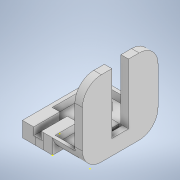
# Autodesk Inventor part: InstaMeter
Saved by Autodesk Inventor 2020 (Build 240168000, 168)
## iProperties
Created: 2020-01-07
Part Number: InstaMeter
Material: Générique
Document SubType Name: Modeling
Designer: laura
Density: 1 g/cm^3
Appearance: Par défaut
Author: laura
## iProperties of the stored document _Impression 3D.ipt
Created: 2020-01-09
Part Number: _Impression 3D
Material: Générique
Document SubType Name: Modeling
Designer: laura
Density: 1 g/cm^3
Appearance: Par défaut
Author: laura
Autodesk Inventor part; units mm, degrees
ref_plane "YZ Plane" through (0, 0, 0) normal (1, 0, 0) x (0, 1, 0)
sketch "Esquisse1" plane through (0, 0, 0) normal (0, 1, 0) x (-1, 0, 0)
  line L0 (0, 0) -> (-40, 0)
  line L1 (-40, 0) -> (-40, -80)
  line L2 (-40, -80) -> (0, -80)
  line L3 (0, -80) -> (0, 0)
  dimension "d0" = 80
  dimension "d4" = 40
  constraints: 8 end point, 2 parallel, 1 horizontal, 1 perpendicular
  measures "d0" distance between parallel lines of L2 L0
  measures "d4" distance between parallel lines of L1 L3
extrude "Extrusion1" add sketch "Esquisse1" along normal blind 80
sketch "Esquisse2" plane through (40, 0, 0) normal (1, 0, 0) x (0, 0, -1)
  point P0 (0, 0)
sketch "Esquisse3" plane through (40, 0, 0) normal (1, 0, 0) x (0, 0, -1)
  line L0 (0, 80) -> (80, 80) projected
  line L1 (20, 20) -> (60, 20)
  line L2 (60, 20) -> (60, 80)
  line L3 (60, 80) -> (20, 80)
  line L4 (20, 80) -> (20, 20)
  line L5 (0, 0) -> (80, 0) projected
  line L6 (80, 0) -> (80, 80) projected
  line L7 (0, 0) -> (0, 80) projected
  point P0 (20, 80)
  dimension "d9" = 20
  dimension "d10" = 20
  dimension "d11" = 20
  constraints: 8 end point, 2 parallel, 1 horizontal, 1 perpendicular, 1 point on line
  measures "d9" distance between parallel lines of L5 L1
  measures "d10" distance between parallel lines of L6 L2
  measures "d11" distance between parallel lines of L7 L4
extrude "Extrusion2" cut sketch "Esquisse3" against normal blind 80 contours L0 L2 L1 L4
sketch "Esquisse4" plane through (40, 20, -20) normal (0, 1, 0) x (1, 0, 0)
  line L0 (0, 40) -> (-40, 40) projected
  line L1 (0, 0) -> (-5, 0)
  line L2 (-5, 40) -> (0, 40)
  line L3 (0, 40) -> (0, 0)
  line L4 (-5, 40) -> (-10, 40)
  line L5 (-9, 10) -> (-12, 10)
  line L6 (-12, 10) -> (-12, 30)
  line L7 (-12, 30) -> (-9, 30)
  line L8 (-9, 10) -> (-9, 30)
  point P0 (-40, -20)
  dimension "d19" = 20
  dimension "d21" = 9
  dimension "d22" = 3
  constraints: 16 end point, 2 horizontal, 2 vertical, 1 parallel, 1 point on line
  measures "d19" distance of L5.end L6.end
  measures "d21" distance between parallel lines of L8 L3
  measures "d22" distance of L5.start L5.end
extrude "Extrusion3" cut sketch "Esquisse4" against normal blind 10
sketch "Esquisse6" plane through (40, 20, -20) normal (0, 0, -1) x (-1, 0, 0)
  line L0 (40, 60) -> (40, 0) projected
  line L1 (0, 60) -> (40, 60) projected
  line L2 (0, 0) -> (0, 60) projected
  line L3 (0, 0) -> (40, 0) projected
  point P0 (40, -20)
extrude "Extrusion4" add sketch "Esquisse6" along normal blind 9
sketch "Esquisse7" plane through (40, 20, -60) normal (0, 0, 1) x (1, 0, 0)
  line L0 (-40, 0) -> (-40, 60) projected
  line L1 (0, 0) -> (-40, 0) projected
  line L2 (0, 60) -> (0, 0) projected
  line L3 (-40, 60) -> (0, 60) projected
  point P0 (-40, -20)
extrude "Extrusion5" add sketch "Esquisse7" along normal blind 9
sketch "Esquisse8" plane through (0, 80, 0) normal (0, 1, 0) x (1, 0, 0)
  line L0 (40, 51) -> (40, 80) projected
  line L1 (40, 80) -> (0, 80) projected
  line L2 (0, 80) -> (0, 51) projected
  line L3 (40, 51) -> (0, 51) projected
  point P0 (0, 0)
extrude "Extrusion6" add sketch "Esquisse8" along normal blind 20
sketch "Esquisse9" plane through (0, 80, 0) normal (0, 1, 0) x (1, 0, 0)
  line L0 (0, 29) -> (0, 0) projected
  line L1 (0, 0) -> (40, 0) projected
  line L2 (40, 0) -> (40, 29) projected
  line L3 (0, 29) -> (40, 29) projected
extrude "Extrusion7" add sketch "Esquisse9" along normal blind 20
sketch "Esquisse10" plane through (0, 0, 0) normal (0, 0, 1) x (1, 0, 0)
  line L0 (0, 0) -> (40, 0) projected
  line L1 (40, 0) -> (40, 100) projected
  line L2 (0, 100) -> (40, 100) projected
  line L3 (0, 0) -> (0, 100) projected
extrude "Extrusion8" add sketch "Esquisse10" along normal blind 10
sketch "Esquisse11" plane through (40, 0, -80) normal (0, 0, -1) x (-1, 0, 0)
  line L0 (0, 0) -> (40, 0) projected
  line L1 (40, 0) -> (40, 100) projected
  line L2 (0, 100) -> (40, 100) projected
  line L3 (0, 0) -> (0, 100) projected
extrude "Extrusion9" add sketch "Esquisse11" along normal blind 10
sketch "Esquisse12" plane through (0, 20, -51) normal (-1, 0, 0) x (0, 0, 1)
  line L0 (22, 80) -> (61, 80) projected
  line L1 (61, 80) -> (36, 80)
  line L2 (61, 80) -> (61, 55)
  line L3 (61, 80) -> (61, -20) projected
  arc A0 (61, 55) -> (36, 80) centre (36, 55) ccw
  point P0 (51, -20)
  dimension "d35" = 25
  dimension "d36" = 25
  constraints: 4 end point, 2 point on circle, 2 point on line, 1 centre point, 1 tangent
  measures "d35" distance of L0.end L1.end
  measures "d36" distance of L0.end L2.end
ref_plane "Plan de construction1" through (40, 0, -40) normal (0, 0, -1) x (-1, 0, 0)
extrude "Extrusion10" cut sketch "Esquisse12" against normal up to surface (40 mm away)
mirror "Symétrie1" about plane through (40, 0, -40) normal (0, 0, -1) of "Extrusion10"
ref_plane "Plan de construction2" through (0, 50, 0) normal (0, 1, 0) x (1, 0, 0)
mirror "Symétrie2" about plane through (0, 50, 0) normal (0, 1, 0) of "Extrusion10", "Symétrie1"
sketch "Esquisse13" plane through (0, 20, -51) normal (-1, 0, 0) x (0, 0, 1)
  line L0 (11, -10) -> (-14, -10)
  line L1 (11, -10) -> (36, -10)
  line L2 (-14, -10) -> (-14, 0)
  line L3 (-14, 0) -> (-38.4949, 0)
  line L4 (36, -10) -> (36, 0)
  line L5 (36, 0) -> (60.4949, 0)
  arc A0 (-38.4949, 0) -> (-14, -20) centre (-14, 5) ccw
  arc A1 (36, -20) -> (60.4949, 0) centre (36, 5) ccw
  line L6 (36, -20) -> (-14, -20)
  point P0 (51, -20)
  dimension "d40" = 25
  dimension "d41" = 25
  dimension "d42" = 10
  constraints: 14 end point, 4 point on circle, 2 centre point, 2 point on line
  measures "d40" distance of L0.start L0.end
  measures "d41" distance of L0.start L1.end
  measures "d42" distance of L0.end L2.end
extrude "Extrusion11" add sketch "Esquisse13" along normal blind 40
sketch "Esquisse14" plane through (0, 10, -15) normal (0, 1, 0) x (1, 0, 0)
  line L0 (-40, 0) -> (-40, 50) projected
  line L1 (-40, 0) -> (40, 0) projected
  line L2 (-40, 50) -> (-35, 50)
  line L3 (-35, 50) -> (-35, 0)
  line L4 (-35, 0) -> (-40, 0)
  line L5 (-40, 0) -> (-40, 50)
  point P0 (0, -15)
  dimension "d45" = 5
  constraints: 8 end point, 2 parallel, 1 horizontal, 1 perpendicular, 1 point on line
  measures "d45" distance of L3.end L4.end
extrude "Extrusion12" add sketch "Esquisse14" along normal up to surface (10 mm away)
sketch "Esquisse15" plane through (0, 20, 9.4949) normal (0, 1, 0) x (1, 0, 0)
  line L0 (-17.5, 24.4949) -> (-12.5, 24.4949)
  line L1 (-12.5, 24.4949) -> (-22.5, 24.4949)
  line L2 (-22.5, 24.4949) -> (-22.5, 0)
  line L3 (-12.5, 24.4949) -> (-12.5, 0)
  line L4 (-22.5, 0) -> (-12.5, 0)
  dimension "d48" = 5
  dimension "d49" = 10
  constraints: 10 end point, 2 perpendicular, 1 parallel
  measures "d48" distance of L0.start L0.end
  measures "d49" distance of L0.end L1.end
extrude "Extrusion13" cut sketch "Esquisse15" against normal up to surface (10 mm away)
sketch "Esquisse16" plane through (40, 20, -51) normal (0, 0, 1) x (1, 0, 0)
  point P0 (-40, -20)
sketch "Esquisse17" plane through (31, 20, -50) normal (-1, 0, 0) x (0, 0, 1)
  line L0 (0, 0) -> (20, 0) projected
  line L1 (0, 0) -> (0, -10) projected
  line L2 (0, -10) -> (20, -10) projected
  line L3 (20, 0) -> (20, -10) projected
  point P0 (50, -20)
extrude "Extrusion14" cut sketch "Esquisse17" against normal blind 1
sketch "Esquisse18" plane through (0, 20, -51) normal (-1, 0, 0) x (0, 0, 1)
  line L0 (22, 0) -> (22, 80)
  line L1 (22, 80) -> (36, 80)
  arc A0 (61, 55) -> (36, 80) centre (36, 55) ccw
  line L2 (-38.4949, 0) -> (-14, 0)
  line L3 (36, 0) -> (60.4949, 0)
  arc A1 (60.4949, 0) -> (61, 5) centre (36, 5) ccw
  line L4 (61, 55) -> (61, 5)
  arc A2 (61, 55) -> (36, 80) centre (36, 55) ccw
  line L5 (22, 80) -> (36, 80)
  line L6 (22, 0) -> (22, 80)
  line L7 (22, 0) -> (0, 0)
  line L8 (0, 0) -> (0, 80)
  line L9 (0, 80) -> (-14, 80)
  arc A3 (-14, 80) -> (-39, 55) centre (-14, 55) ccw
  line L10 (-39, 5) -> (-39, 55)
  arc A4 (-39, 5) -> (-38.4949, 0) centre (-14, 5) ccw
  arc A5 (-39, 5) -> (-38.4949, 0) centre (-14, 5) ccw
  line L11 (-38.4949, 0) -> (60.4949, 0)
  point P0 (51, -20)
  point P1 (61, 55)
  point P2 (22, 0)
  point P3 (36, 0)
  constraints: 24 end point, 12 point on circle, 10 centre point
extrude "Extrusion15" cut sketch "Esquisse18" against normal blind 30
sketch "Esquisse19" plane through (0, 10, -65) normal (0, 0, 1) x (1, 0, 0)
  line L0 (-35, 10) -> (-35, 0) projected
  line L1 (0, 0) -> (-35, 0) projected
  line L2 (0, 10) -> (0, 0) projected
  line L3 (0, 10) -> (-35, 10) projected
  point P0 (0, -10)
extrude "Extrusion16" cut sketch "Esquisse19" against normal blind 20
sketch "Esquisse20" plane through (0, 10, -15) normal (-1, 0, 0) x (0, 0, 1)
  arc A0 (0, -10) -> (25, 15) centre (0, 15) ccw projected
  line L0 (25, 15) -> (25, -10)
  line L1 (25, -10) -> (0, -10)
  line L2 (24.498, 10.0154) -> (25, 10.0154)
  point P0 (15, -10)
  constraints: 6 end point, 2 perpendicular, 2 tangent, 1 point on circle, 1 point on line, 1 vertical
extrude "Extrusion17" add sketch "Esquisse20" along normal up to surface (40 mm away) contours A0 L2 L0 L1
mirror "Symétrie3" about plane through (40, 0, -40) normal (0, 0, -1) of "Extrusion17"
sketch "Esquisse21" plane through (0, 0, 10) normal (0, 0, 1) x (1, 0, 0)
  line L0 (-22.5, 20) -> (-22.5, 10) projected
  line L1 (-12.5, 10) -> (-12.5, 20) projected
  line L2 (-22.5, 10) -> (-35, 10) projected
  line L3 (-12.5, 10) -> (-22.5, 10) projected
  line L4 (0, 10) -> (-12.5, 10) projected
  line L5 (-35, 10) -> (0, 10) projected
  line L6 (0, 20) -> (-12.5, 20) projected
  line L7 (-22.5, 20) -> (-22.5, 21.5856)
  line L8 (-12.5, 20) -> (-12.5, 21.5856)
  line L9 (-12.5, 21.5856) -> (-22.5, 21.5856)
  point P0 (0, 0)
  point P1 (-22.5, 10)
  point P2 (-12.5, 10)
  constraints: 6 end point, 2 vertical, 1 perpendicular
extrude "Extrusion18" cut sketch "Esquisse21" against normal blind 20
sketch "Esquisse23" plane through (40, 20, -29) normal (0, 1, 0) x (1, 0, 0)
  line L0 (-40, -14) -> (-40, 56)
  line L1 (-10, 0) -> (0, 0)
  line L2 (-8, 22) -> (-10, 22)
  line L3 (-10, 22) -> (-10, 56)
  line L4 (-8, 1) -> (-12, 1)
  line L5 (-12, 21) -> (-8, 21)
  line L6 (-8, 21) -> (-8, 1)
  line L7 (-10, 22) -> (-10, 56)
  line L8 (-10, 22) -> (-40, 22)
  line L9 (-40, -14) -> (-40, 56)
  line L10 (-10, 22) -> (-10, 56)
  line L11 (-40, 56) -> (-10, 56)
  point P0 (-10, -38.4949)
  point P1 (-40, 22)
  constraints: 24 end point, 2 point on line
extrude "Extrusion20" cut sketch "Esquisse23" against normal blind 10
mirror "Symétrie4" about plane through (40, 0, -40) normal (0, 0, -1) of "Extrusion20"
sketch "Esquisse24" plane through (0, 20, 9.4949) normal (0, 1, 0) x (1, 0, 0)
  point P0 (0, 9.4949)
sketch "Esquisse25" plane through (0, 20, 9.4949) normal (0, 1, 0) x (1, 0, 0)
  point P0 (0, 9.4949)
sketch "Esquisse26" plane through (0, 0, 10) normal (0, 0, 1) x (1, 0, 0)
  point P0 (0, 0)
sketch "Esquisse27" plane through (-40, 20.0154, 9.498) normal (0, 1, 0) x (1, 0, 0)
  line L0 (27.5, -0.502) -> (27.5, 24.498) projected
  line L1 (40, 24.498) -> (40, -0.502) projected
  line L2 (27.5, 0.0017) -> (40, 0.0017)
  line L3 (40, 0.0017) -> (40, -0.502)
  line L4 (40, -0.502) -> (27.5, -0.502)
  line L5 (27.5, -0.502) -> (27.5, 0.0017)
  point P0 (40, 9.498)
  constraints: 8 end point, 2 parallel, 1 horizontal, 1 perpendicular, 1 point on line
extrude "Extrusion21" cut sketch "Esquisse27" against normal blind 25
sketch "Esquisse28" plane through (-40, 20.0154, 9.498) normal (0, 1, 0) x (1, 0, 0)
  point P0 (40, 9.498)
sketch "Esquisse29" plane through (-40, 20.0154, 9.498) normal (0, 1, 0) x (1, 0, 0)
  line L0 (17.5, -0.502) -> (17.5, 0) projected
  line L1 (17.5, 0) -> (0, 0) projected
  line L2 (0, 0) -> (0, -0.502) projected
  line L3 (17.5, -0.502) -> (0, -0.502) projected
  point P0 (40, 9.498)
extrude "Extrusion22" cut sketch "Esquisse29" against normal up to surface (20.0154 mm away)
sketch "Esquisse30" plane through (-35, 10, -15) normal (0, 1, 0) x (1, 0, 0)
  line L0 (22.5, -25) -> (12.5, -25) projected
  line L1 (12.5, -25) -> (12.5, -24.4949)
  line L2 (22.5, -24.4963) -> (22.5, 0) projected
  line L3 (12.5, -24.4949) -> (22.5, -24.4963)
  line L4 (22.5, -25) -> (22.5, -24.4963) projected
  line L5 (22.5, -24.4963) -> (22.5, -25)
  point P0 (35, -15)
  constraints: 6 end point, 1 vertical
extrude "Extrusion23" cut sketch "Esquisse30" against normal up to surface (10 mm away)
sketch "Esquisse31" plane through (-40, 20.0154, -89.498) normal (0, 1, 0) x (1, 0, 0)
  line L0 (0, 0) -> (0, 0.502) projected
  line L1 (40, 0) -> (0, 0) projected
  line L2 (40, 0.502) -> (40, 0) projected
  line L3 (40, 0.502) -> (0, 0.502) projected
  point P0 (40, -89.498)
extrude "Extrusion24" cut sketch "Esquisse31" against normal up to surface (20.0154 mm away)
sketch "Esquisse32" plane through (0, 10, -51) normal (-1, 0, 0) x (0, 0, 1)
  line L0 (0, 0) -> (0, 10)
  line L1 (0, 10) -> (22, 10)
  line L2 (22, 10) -> (22, 0)
  line L3 (22, 0) -> (0, 0)
  point P0 (51, -10)
  constraints: 8 end point, 2 parallel, 1 perpendicular, 1 vertical
extrude "Extrusion25" add sketch "Esquisse32" along normal blind 5
sketch "Esquisse37" plane through (-35, 20, -15) normal (0, 1, 0) x (1, 0, 0)
  line L0 (12.5, 0) -> (0, 0) projected
  line L1 (12.5, 0) -> (10, 0)
  line L2 (10, 0) -> (10, -25.2265)
  line L3 (10, -25.2265) -> (12.5, -25.2265)
  line L4 (12.5, -25.2265) -> (12.5, 0)
  point P0 (35, -15)
  dimension "d78" = 2.5
  constraints: 8 end point, 2 parallel, 1 horizontal, 1 perpendicular
  measures "d78" distance of L3.end L2.end
extrude "Extrusion27" cut sketch "Esquisse37" against normal blind 10
sketch "Esquisse39" plane through (0, 20, 9.4949) normal (0, 1, 0) x (1, 0, 0)
  line L0 (-12.5, 24.4949) -> (-12.5, 0) projected
  line L1 (-12.5, 24.4949) -> (-12.5, 0)
  line L2 (-12.5, 0) -> (-15, 0)
  line L3 (-15, 0) -> (-15, 24.4949)
  line L4 (-15, 24.4949) -> (-12.5, 24.4949)
  point P0 (0, 9.4949)
  dimension "d81" = 2.5
  constraints: 8 end point, 2 parallel, 1 perpendicular, 1 vertical
  measures "d81" distance of L0.end L2.end
extrude "Extrusion28" add sketch "Esquisse39" against normal blind 10
sketch "Esquisse40" plane through (-35, 10, -15) normal (0, 1, 0) x (1, 0, 0)
  line L0 (30, 14) -> (30, 36) projected
  line L1 (30, 14) -> (30, 0)
  line L2 (35, 0) -> (20, 0) projected
  line L3 (35, -20) -> (35, 0) projected
  line L4 (35, -20) -> (35, 0)
  line L5 (35, 0) -> (30, 0)
  line L6 (30, 0) -> (30, -20)
  line L7 (30, -20) -> (35, -20)
  point P0 (35, -15)
  point P1 (30, 0)
  constraints: 10 end point, 3 equal length, 1 perpendicular, 1 point on line, 1 vertical
extrude "Extrusion29" cut sketch "Esquisse40" along normal blind 10
sketch "Esquisse41" plane through (-15, 10, -15) normal (0, 0, -1) x (-1, 0, 0)
  line L0 (-10, 10) -> (-10, 0) projected
  line L1 (-10, 10) -> (0, 10) projected
  line L2 (-10, 0) -> (-10, 10)
  line L3 (-10, 10) -> (0, 10)
  line L4 (0, 10) -> (0, 0)
  line L5 (0, 0) -> (-10, 0)
  point P0 (-15, -10)
  constraints: 8 end point, 2 parallel, 1 perpendicular, 1 vertical
extrude "Extrusion30" add sketch "Esquisse41" along normal blind 10
sketch "Esquisse42" plane through (0, 20, 9.4949) normal (0, 1, 0) x (1, 0, 0)
  point P0 (0, 9.4949)
sketch "Esquisse43" plane through (-35, 10, -15) normal (0, 0, -1) x (-1, 0, 0)
  point P0 (-35, -10)
sketch "Esquisse44" plane through (-35, 10, -15) normal (0, 0, -1) x (-1, 0, 0)
  line L0 (-10, 0) -> (0, 0) projected
  line L1 (-10, 10) -> (0, 10) projected
  line L2 (-10, 0) -> (-10, 10)
  line L3 (-10, 10) -> (0, 10)
  line L4 (0, 10) -> (0, 0)
  line L5 (0, 0) -> (-10, 0)
  point P0 (-35, -10)
  constraints: 8 end point, 2 parallel, 1 perpendicular, 1 vertical
extrude "Extrusion31" add sketch "Esquisse44" along normal blind 10
sketch "Esquisse45" plane through (30, 10, -51) normal (0, 0, -1) x (-1, 0, 0)
  line L0 (0, 10) -> (35, 10) projected
  line L1 (35, 10) -> (35, 0) projected
  line L2 (35, 10) -> (35, 0)
  line L3 (35, 0) -> (31.1961, 0)
  line L4 (31.1961, 0) -> (31.1961, 10)
  line L5 (31.1961, 10) -> (35, 10)
  point P0 (30, -10)
  constraints: 8 end point, 3 equal length, 1 perpendicular
extrude "Extrusion32" add sketch "Esquisse45" along normal blind 20 and the other way blind 60
sketch "Esquisse46" plane through (-40, 20.0154, 9.498) normal (0, 0, 1) x (1, 0, 0)
  line L0 (17.5, 0) -> (17.5, -0.0154) projected
  line L1 (17.5, -0.0154) -> (17.5, 0)
  line L2 (17.5, 0) -> (15.0008, 0)
  line L3 (15.0008, 0) -> (15.0008, -0.0154)
  line L4 (15.0008, -0.0154) -> (17.5, -0.0154)
  point P0 (40, -20.0154)
  constraints: 8 end point, 2 parallel, 1 perpendicular, 1 vertical
extrude "Extrusion33" cut sketch "Esquisse46" against normal blind 1
sketch "Esquisse47" plane through (-12.5, 20.0069, 9.4963) normal (0, 0, 1) x (1, 0, 0)
  point P0 (12.5, -20.0069)
ref_plane "Plan de construction3" through (40, 0, -40) normal (0, 0, -1) x (-1, 0, 0)
